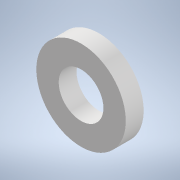
# Autodesk Inventor part: ring
Saved by Autodesk Inventor 2022 (Build 260153000, 153)
## iProperties
Created: 2025-06-24
Part Number: ring
Material: Типовые
Document SubType Name: Modeling
Designer: korsh524
Density: 1 g/cm^3
Appearance: По умолчанию
Author: korsh524
Autodesk Inventor part; units mm, degrees
ref_plane "YZ Plane" through (0, 0, 0) normal (1, 0, 0) x (0, 1, 0)
ref_plane "XZ Plane" through (0, 0, 0) normal (0, 1, 0) x (-1, 0, 0)
ref_plane "XY Plane" through (0, 0, 0) normal (0, 0, 1) x (1, 0, 0)
sketch "Эскиз1" plane through (0, 0, 0) normal (0, 0, 1) x (1, 0, 0)
  arc A0 (49.04, -63.7734) -> (53.3569, -60.2081) centre (57.3118, -69.3928) ccw projected
  circle A1 centre (57.3118, -69.3928) radius 5
  circle A2 centre (57.3118, -69.3928) radius 10
  point P0 (0, 0)
  dimension "d0" = 10
  constraints: 2 coincident, 1 centre point, 3 other
  measures "d0" diameter of A1
extrude "Выдавливание1" add sketch "Эскиз1" along normal blind 4
